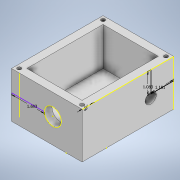
# Autodesk Inventor part: Water_Proof_Box_Bottom
Saved by Autodesk Inventor 2022 (Build 260153000, 153)
## iProperties
Created: 2023-07-12
Part Number: Water_Proof_Box_Bottom
Material: Generic
Document SubType Name: Modeling
Designer: jtw4137
Density: 1 g/cm^3
Appearance: Default
Author: jtw4137
Autodesk Inventor part; units mm, degrees
ref_plane "YZ Plane" through (0, 0, 0) normal (1, 0, 0) x (0, 1, 0)
ref_plane "XZ Plane" through (0, 0, 0) normal (0, 1, 0) x (-1, 0, 0)
ref_plane "XY Plane" through (0, 0, 0) normal (0, 0, 1) x (1, 0, 0)
sketch "Sketch1" plane through (0, 0, 0) normal (0, 1, 0) x (-1, 0, 0)
  line L0 (71.7038, 31.922) -> (71.7038, -88.078)
  line L1 (71.7038, -88.078) -> (-20.7962, -88.078)
  line L2 (-20.7962, -88.078) -> (-20.7962, 31.922)
  line L3 (-20.7962, 31.922) -> (71.7038, 31.922)
  point P0 (0, 0)
  dimension "d0" = 120
  dimension "d1" = 92.5
  constraints: 8 end point, 2 perpendicular, 1 vertical
  measures "d0" distance of L0.start L0.end
  measures "d1" distance of L2.end L0.start
extrude "Extrusion1" add sketch "Sketch1" along normal blind 60
shell "Shell2" thickness 10 removed faces 1 at (-10.0371, 60, -48.078)
sketch "Sketch12" plane through (0, 60, 0) normal (0, 1, 0) x (1, 0, 0)
  line L0 (10.7962, 78.078) -> (10.7962, -21.922) projected
  line L1 (10.7962, -21.922) -> (20.7962, -21.922)
  line L2 (20.7962, -31.922) -> (20.7962, 88.078) projected
  line L3 (20.7962, -21.922) -> (20.7962, -31.922)
  line L4 (20.7962, -31.922) -> (10.7962, -31.922)
  line L5 (10.7962, -31.922) -> (10.7962, -21.922)
  line L6 (20.7962, -31.922) -> (15.8432, -31.922)
  line L7 (-71.7038, -31.922) -> (20.7962, -31.922) projected
  line L8 (15.8432, -26.969) -> (20.7962, -26.969)
  line L9 (15.8432, -26.969) -> (15.8432, -31.922)
  point P0 (0, 0)
  dimension "d124" = 4.953
  dimension "d125" = 4.953
  constraints: 14 end point, 5 perpendicular, 2 point on line, 1 horizontal
  measures "d124" distance of L8.start L6.end
  measures "d125" distance of L8.start L8.end
hole "Hole11" at (15.8432, 60, 26.969) direction (0, -1, 0) diameter 5 depth 25.4 tip angle 118
sketch "Sketch19" plane through (0, 60, 0) normal (0, 1, 0) x (1, 0, 0)
  line L0 (10.7962, -21.922) -> (-61.7038, -21.922) projected
  line L1 (-61.7038, -21.922) -> (-61.7038, -31.922)
  line L2 (-71.7038, -31.922) -> (20.7962, -31.922) projected
  line L3 (-71.7038, -31.922) -> (-71.7038, -21.922)
  line L4 (-71.7038, 88.078) -> (-71.7038, -31.922) projected
  line L5 (-61.7038, -23.8125) -> (-61.7038, -21.922)
  line L6 (-71.7038, -21.922) -> (-61.7038, -21.922)
  line L7 (-61.7038, -21.922) -> (-61.7038, 78.078) projected
  line L8 (-61.7038, -21.922) -> (-66.7038, -21.922)
  line L9 (-66.6566, -26.875) -> (-61.7038, -26.922)
  line L10 (-66.6566, -26.875) -> (-66.7038, -21.922)
  point P0 (0, 0)
  dimension "d133" = 4.953
  dimension "d134" = 4.953
  constraints: 14 end point, 3 point on line, 2 midpoint, 1 parallel, 1 perpendicular, 1 vertical
  measures "d133" distance of L9.start L9.end
  measures "d134" vertical distance of L9.start L8.end
hole "Hole12" at (-66.6566, 60, 26.875) direction (0, -1, 0) diameter 5 depth 25.4 tip angle 118
sketch "Sketch21" plane through (0, 60, 0) normal (0, 1, 0) x (1, 0, 0)
  line L0 (10.7962, -21.922) -> (10.7962, 78.078) projected
  line L1 (10.7962, 78.078) -> (20.7962, 78.078)
  line L2 (20.7962, -31.922) -> (20.7962, 88.078) projected
  line L3 (20.7962, 88.078) -> (10.7962, 88.078)
  line L4 (20.7962, 88.078) -> (-71.7038, 88.078) projected
  line L5 (10.7962, 78.078) -> (10.7962, 88.078)
  line L6 (10.7962, 78.078) -> (-61.7038, 78.078) projected
  line L7 (10.7962, 78.078) -> (15.7962, 78.078)
  line L8 (15.8432, 83.031) -> (20.7962, 83.031)
  line L9 (15.8432, 83.031) -> (15.7962, 78.078)
  point P0 (0, 0)
  dimension "d146" = 4.953
  constraints: 12 end point, 3 point on line, 2 perpendicular, 1 horizontal, 1 midpoint
  measures "d146" distance of L8.start L8.end
hole "Hole13" at (15.8432, 60, -83.031) direction (0, -1, 0) diameter 5 depth 25.4 tip angle 118
sketch "Sketch22" plane through (0, 60, 0) normal (0, 1, 0) x (1, 0, 0)
  line L0 (-61.7038, 78.078) -> (10.7962, 78.078) projected
  line L1 (-61.7038, 78.078) -> (-71.7038, 78.078)
  line L2 (-71.7038, 88.078) -> (-71.7038, -31.922) projected
  line L3 (-71.7038, 88.078) -> (-61.7038, 88.078)
  line L4 (20.7962, 88.078) -> (-71.7038, 88.078) projected
  line L5 (-61.7038, 78.078) -> (-61.7038, 88.078)
  line L6 (-61.7038, 78.078) -> (-66.7038, 78.078)
  line L7 (-66.6568, 83.031) -> (-61.7038, 83.031)
  line L8 (-66.6568, 83.031) -> (-66.7038, 78.078)
  point P0 (0, 0)
  dimension "d155" = 4.953
  dimension "d156" = 4.953
  constraints: 12 end point, 3 point on line, 2 perpendicular, 1 horizontal, 1 midpoint
  measures "d155" distance of L7.start L7.end
  measures "d156" vertical distance of L7.start L6.end
hole "Hole14" at (-66.6568, 60, -83.031) direction (0, -1, 0) diameter 5 depth 25.4 tip angle 118
sketch "Sketch23" plane through (-71.7038, 0, 31.922) normal (0, 0, 1) x (1, 0, 0)
  point P0 (71.7038, 0)
sketch "Sketch24" plane through (-71.7038, 0, 31.922) normal (0, 0, 1) x (1, 0, 0)
  line L0 (0, 0) -> (0, 60) projected
  line L1 (0, 60) -> (0, 0)
  line L2 (0, 0) -> (92.5, 0) projected
  line L3 (0, 0) -> (92.5, 0)
  line L4 (92.5, 0) -> (92.5, 60) projected
  line L5 (92.5, 0) -> (92.5, 60)
  line L6 (0, 60) -> (92.5, 60) projected
  line L7 (92.5, 60) -> (0, 60)
  line L8 (0, 32.5045) -> (54, 32.5045)
  line L9 (54, 32.5045) -> (46.25, 60)
  line L10 (82.5, 60) -> (10, 60) projected
  point P0 (71.7038, 0)
  dimension "d164" = 60
  dimension "d165" = 92.5
  dimension "d175" = 54
  dimension "d176" = 27.4955
  constraints: 12 end point, 3 collinear, 2 perpendicular, 1 midpoint, 1 point on line
  measures "d164" distance of L0.start L0.end
  measures "d165" distance of L0.end L4.end
  measures "d175" distance of L8.start L8.end
  measures "d176" vertical distance of L8.end L9.end
hole "Hole15" at (-17.7038, 32.5045, 31.922) direction (0, 0, -1) diameter 22 depth 25.4 tip angle 118
sketch "Sketch32" plane through (20.7962, 0, 31.922) normal (1, 0, 0) x (0, 0, -1)
  line L0 (0, 60) -> (120, 60) projected
  line L1 (90, 60) -> (90, 32.5)
  line L2 (90, 32.5) -> (120, 32.5)
  line L3 (120, 0) -> (120, 60) projected
  point P0 (31.922, 0)
  dimension "d189" = 27.5
  dimension "d190" = 30
  constraints: 4 end point, 2 perpendicular, 2 point on line
  measures "d189" distance of L1.start L1.end
  measures "d190" distance of L1.end L2.end
sketch "Sketch33" plane through (20.7962, 0, 31.922) normal (1, 0, 0) x (0, 0, -1)
  line L0 (89.9856, 20.7094) -> (89.9856, 34.3094) construction
  line L1 (82.4856, 28.2094) -> (82.4856, 26.8094)
  line L2 (97.4856, 26.8094) -> (97.4856, 28.2094)
  arc A0 (82.4856, 28.2094) -> (97.4856, 28.2094) centre (89.9856, 28.2094) ccw
  arc A1 (97.4856, 26.8094) -> (82.4856, 26.8094) centre (89.9856, 26.8094) ccw
  point P0 (31.922, 0)
  point P1 (89.9856, 27.5094)
  point P2 (97.4528, 27.5094)
  point P3 (82.5183, 27.5094)
  dimension "d191" = 13.6
  dimension "d192" = 7.5
  constraints: 8 end point, 6 point on circle, 4 tangent, 2 centre point, 2 point on line, 1 midpoint, 1 parallel, 1 vertical
  measures "d191" distance of L0.start L0.end
  measures "d192" distance from line of L2 point (89.986, 27.509)
extrude "Extrusion2" cut sketch "Sketch33" against normal blind 10 contours A1 A0
sketch "Sketch35" plane through (-71.7038, 0, 31.922) normal (0, 0, 1) x (1, 0, 0)
  circle A0 centre (54, 32.5045) radius 11 projected
  line L0 (43, 32.5045) -> (-0.012, 32.5045)
  line L1 (10, 10) -> (10, 60) projected
  point P0 (71.7038, 0)
  dimension "d195" = 43.012
  constraints: 2 end point, 1 horizontal alignment, 1 perpendicular, 1 other
  measures "d195" distance of L0.start L0.end
body "Solid1"
